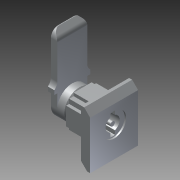
# Autodesk Inventor part: 1XXX_01_05_1
Saved by Autodesk Inventor 2016 (Build 200138000, 138)
## iProperties
Category: PARTsolutions
Company: RITTAL
Created: 2014-04-04
Part Number: 1XXX_01_05_1
Catalog Web Link: www.cadenas.de
Description: Vorreiberverschluss AE-Vorreiberverschluss AE
Vendor: RITTAL
Document SubType Name: Modeling
Designer: PARTuser1
Manufacturer: RITTAL
Density: 1 g/cm^3
Material: Generic
Appearance: RGB(195.00000357627781,201.00000321865156,196.00000351667384)
PSOL_IDENT_0: {$CADENAS_DATA\23d-libs\rittal\schaltschranksys\kompakt_schaltschr\ae\parts_ae\vorreiberverschluss_a
PSOL_IDENT_1: e.prj},188 {VTYP=3D},{NB=1XXX_01_05_1},{LINA=1XXX_01_05_1},{NN=Vorreiberverschluss AE},{DATE=26.03.2
PSOL_IDENT_2: 014 14:46:13},{GEOMDATE=26.03.2014 14:45:00},{VERSION=},{LINEID=10},{LINESUBID=-1},{WBVAR=DETAIL}  {
PSOL_IDENT_3: NB=1XXX_01_05_1},{LINA=1XXX_01_05_1},{KT=DUMMY},{BEST=1XXX},{VERS=1},{DETAIL=1}
CNS_NN: Vorreiberverschluss AE
CNS_NT: Vorreiberverschluss AE
CNS_NB: 1XXX_01_05_1
CNS_NBSYN: $BEST._01_05_$DETAIL.
CNS_LINA: 1XXX_01_05_1
CNS_BEST: 1XXX
CNS_VERS: 1
CNS_DETAIL: 1
SUPPLIER: RITTAL
ARTICLENO: 1XXX_01_05_1
BOMINFO: 1XXX_01_05_1
CREATOR: CADENAS GmbH
Title: 1XXX_01_05_1
Author: Cadenas PARTsolutions
Comments: Vorreiberverschluss AE
Autodesk Inventor part; units mm, degrees
sketch "Sketch_1" plane through (0, 0, 0) normal (0, 1, 0) x (-1, 0, 0)
  line L0 (0, 16) -> (-2, 16)
  line L1 (-2, 16) -> (-6, 12)
  line L2 (-6, 12) -> (-6, -20)
  line L3 (-6, -20) -> (-4, -20)
  line L4 (-4, -20) -> (0, -16)
  line L5 (0, -16) -> (0, 16)
  constraints: 12 end point
extrude "Extrusion1" add sketch "Sketch_1" along normal mid plane 32
sketch "Sketch_2" plane through (0, 0, 0) normal (1, 0, 0) x (0, 1, 0)
  line L0 (15, 15) -> (-15, 15)
  line L1 (-15, 15) -> (-15, -15)
  line L2 (-15, -15) -> (15, -15)
  line L3 (15, -15) -> (15, 15)
  constraints: 8 end point
extrude "Extrusion2" add sketch "Sketch_2" against normal blind 1
sketch "Sketch_3" plane through (0, 0, 0) normal (1, 0, 0) x (0, 1, 0)
  line L0 (11, 11) -> (-11, 11)
  line L1 (-11, 11) -> (-11, -11)
  line L2 (-11, -11) -> (11, -11)
  line L3 (11, -11) -> (11, 11)
  constraints: 8 end point
extrude "Extrusion3" cut sketch "Sketch_3" along normal mid plane 3
sketch "Sketch_5" plane through (0, 0, 0) normal (0, 1, 0) x (-1, 0, 0)
  line L0 (15, -9) -> (15, 9)
  line L1 (15, 9) -> (-1.5, 9)
  line L2 (-1.5, 9) -> (-1.5, -9)
  line L3 (-1.5, -9) -> (15, -9)
  constraints: 8 end point
extrude "Extrusion4" add sketch "Sketch_5" along normal mid plane 18
sketch "Sketch_4" plane through (0, 0, 0) normal (0, 1, 0) x (-1, 0, 0)
  line L0 (15, -6) -> (15, 6)
  line L1 (15, 6) -> (-1.5, 6)
  line L2 (-1.5, 6) -> (-1.5, -6)
  line L3 (-1.5, -6) -> (15, -6)
  constraints: 8 end point
extrude "Extrusion5" add sketch "Sketch_4" along normal mid plane 22
sketch "Sketch_7" plane through (0, 0, 0) normal (0, 0, 1) x (1, 0, 0)
  line L0 (-15, 6) -> (-15, -6)
  line L1 (-15, -6) -> (1.5, -6)
  line L2 (1.5, -6) -> (1.5, 6)
  line L3 (1.5, 6) -> (-15, 6)
  constraints: 8 end point
extrude "Extrusion6" add sketch "Sketch_7" along normal mid plane 22
sketch "Sketch_10" plane through (0, 0, 0) normal (0, 0, 1) x (1, 0, 0)
  line L0 (-15, 0) -> (-20.45, 0)
  line L1 (-20.45, 0) -> (-26.2, 5.75)
  line L2 (-26.2, 5.75) -> (-26.2, 10)
  line L3 (-26.2, 10) -> (-17.2, 10)
  line L4 (-17.2, 10) -> (-16.2, 9)
  line L5 (-16.2, 9) -> (-16.2, 5)
  line L6 (-16.2, 5) -> (-15, 5)
  line L7 (-15, 5) -> (-15, 0)
  line L8 (-15, 0) -> (-20.45, 0)
  constraints: 18 end point
revolve "Revolution1" add sketch "Sketch_10" angle 360 about axis through (-15, 0, 0) along (1, 0, 0)
sketch "Sketch_11" plane through (0, 0, 0) normal (0, 0, 1) x (1, 0, 0)
  line L0 (-20.4, 0) -> (-26.2, 0)
  line L1 (-25.7, 0) -> (-25.7, 4.65)
  line L2 (-25.7, 4.65) -> (-25.05, 4.65)
  line L3 (-25.05, 4.65) -> (-20.4, 0)
  line L4 (-20.4, 0) -> (-25.7, 0)
  constraints: 10 end point
revolve "Revolution2" add sketch "Sketch_11" angle 360 about axis through (-20.4, 0, 0) along (1, 0, 0)
sketch "Sketch_12" plane through (-25.7, 0, 0) normal (1, 0, 0) x (0, 0, -1)
  line L0 (-2.65, 0.4) -> (-2.65, -0.4)
  line L1 (-2.65, -0.4) -> (-0.4, -0.4)
  line L2 (-0.4, -0.4) -> (-0.4, -2.65)
  line L3 (-0.4, -2.65) -> (0.4, -2.65)
  line L4 (0.4, -2.65) -> (0.4, -0.4)
  line L5 (0.4, -0.4) -> (2.65, -0.4)
  line L6 (2.65, -0.4) -> (2.65, 0.4)
  line L7 (2.65, 0.4) -> (0.4, 0.4)
  line L8 (0.4, 0.4) -> (0.4, 2.65)
  line L9 (0.4, 2.65) -> (-0.4, 2.65)
  line L10 (-0.4, 2.65) -> (-0.4, 0.4)
  line L11 (-0.4, 0.4) -> (-2.65, 0.4)
  constraints: 24 end point
extrude "Extrusion7" cut sketch "Sketch_12" along normal blind 3
sketch "Sketch_13" plane through (-26.2, 0, 0) normal (1, 0, 0) x (0, 0, -1)
  arc A0 (-44, -5) -> (-39, -10) centre (-39, -5) ccw
  line L0 (-39, -10) -> (-16, -10)
  arc A1 (-12, -12) -> (-16, -10) centre (-16, -15) ccw
  line L1 (-12, -12) -> (-9.2, -12)
  line L2 (-9.2, -12) -> (-9.2, -10)
  line L3 (-9.2, -10) -> (0, -10)
  line L4 (0, -10) -> (0, -6)
  arc A2 (0, 6) -> (0, -6) centre (0, 0) ccw
  line L5 (0, 6) -> (0, 10)
  line L6 (0, 10) -> (-9.2, 10)
  line L7 (-9.2, 10) -> (-9.2, 12)
  line L8 (-9.2, 12) -> (-12, 12)
  arc A3 (-16, 10) -> (-12, 12) centre (-16, 15) ccw
  line L9 (-16, 10) -> (-39, 10)
  arc A4 (-39, 10) -> (-44, 5) centre (-39, 5) ccw
  line L10 (-44, 5) -> (-44, -5)
  constraints: 22 end point, 10 point on circle, 5 centre point
extrude "Extrusion8" add sketch "Sketch_13" along normal blind 4.3
sketch "Sketch_14" plane through (0, 0, 0) normal (0, 1, 0) x (-1, 0, 0)
  line L0 (28, 34) -> (28, 49)
  line L1 (28, 49) -> (18, 49)
  line L2 (18, 49) -> (18, 34)
  line L3 (18, 34) -> (21.9, 34)
  line L4 (21.9, 34) -> (21.9, 38.5431)
  arc A0 (23.0716, 41.3716) -> (21.9, 38.5431) centre (25.9, 38.5431) ccw
  line L5 (23.0716, 41.3716) -> (25.7, 44)
  line L6 (25.7, 44) -> (26.2, 44)
  line L7 (26.2, 44) -> (26.2, 34)
  line L8 (26.2, 34) -> (28, 34)
  constraints: 18 end point, 2 point on circle, 1 centre point
extrude "Extrusion9" cut sketch "Sketch_14" along normal mid plane 20
sketch "Sketch_15" plane through (-4.2, 0, 0) normal (1, 0, 0) x (0, 0, -1)
  circle A0 centre (0, 0) radius 8
  constraints: 1 centre point
extrude "Extrusion10" cut sketch "Sketch_15" along normal blind 10.2
sketch "Sketch_16" plane through (-4.2, 0, 0) normal (1, 0, 0) x (0, 0, -1)
  circle A0 centre (0, 0) radius 8
  arc A1 (-7.0931, 1.5) -> (-7.0931, -1.5) centre (0, 0) ccw
  line L0 (-7.0931, -1.5) -> (-4.4542, -1.5)
  arc A2 (-4.4542, -1.5) -> (4.4542, -1.5) centre (0, 0) ccw
  line L1 (4.4542, -1.5) -> (7.0931, -1.5)
  arc A3 (7.0931, -1.5) -> (7.0931, 1.5) centre (0, 0) ccw
  line L2 (7.0931, 1.5) -> (4.4542, 1.5)
  arc A4 (4.4542, 1.5) -> (-4.4542, 1.5) centre (0, 0) ccw
  line L3 (-4.4542, 1.5) -> (-7.0931, 1.5)
  constraints: 8 end point, 8 point on circle, 5 centre point
extrude "Extrusion11" add sketch "Sketch_16" along normal blind 9.2
sketch "Sketch_17" plane through (0, 0, 0) normal (1, 0, 0) x (0, 1, 0)
  circle A0 centre (0, 0) radius 1.5
  constraints: 1 centre point
extrude "Extrusion12" add sketch "Sketch_17" along normal mid plane 10
ref_plane "verschluss_XY" through (-1, 0, 0) normal (1, 0, 0) x (0, 0, -1)
ref_plane "verschluss_YZ" through (-1, 0, 0) normal (0, 0, -1) x (0, 1, 0)
ref_plane "verschluss_ZX" through (-1, 0, 0) normal (0, 1, 0) x (1, 0, 0)
body "Solid1"
